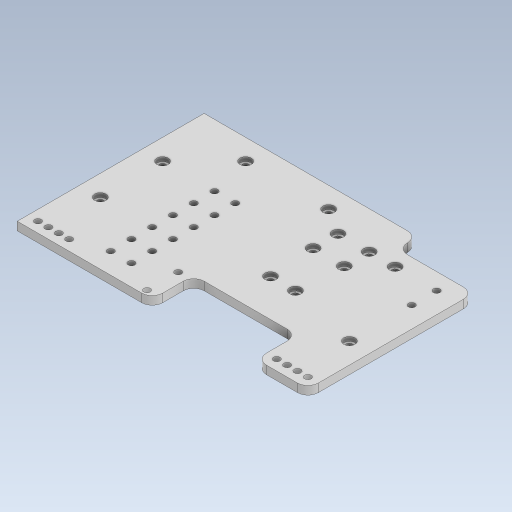
# Autodesk Inventor part: Fix Casis Kiri Belakang
Saved by Autodesk Inventor 2023.5 (Build 275446000, 446)
## iProperties
Created: 2025-10-01
Part Number: Fix Casis Kiri Belakang
Material: Generic
Document SubType Name: Modeling
Designer: Guntur
Density: 1 g/cm^3
Appearance: Default
Author: Guntur
## iProperties of the stored document Fix Casis Kiri Belakang_3DPrint.ipt
Created: 2025-10-18
Part Number: Fix Casis Kiri Belakang_3DPrint
Material: Generic
Document SubType Name: Modeling
Designer: Guntur
Density: 1 g/cm^3
Appearance: Default
Author: Guntur
Autodesk Inventor part; units mm, degrees
ref_plane "YZ Plane" through (0, 0, 0) normal (1, 0, 0) x (0, 1, 0)
ref_plane "XZ Plane" through (0, 0, 0) normal (0, 1, 0) x (-1, 0, 0)
ref_plane "XY Plane" through (0, 0, 0) normal (0, 0, 1) x (1, 0, 0)
sketch "Sketch1" plane through (0, 0, 0) normal (0, 1, 0) x (-1, 0, 0)
  circle A0 centre (-125, -5) radius 1.6
  circle A1 centre (-120, -5) radius 1.6
  line L0 (-115, -20) -> (-115, 0)
  line L1 (-115, 0) -> (-65, 0)
  line L2 (-65, -20) -> (-115, -20)
  line L3 (-65, 0) -> (-65, -20)
  circle A2 centre (-130, -5) radius 1.6
  circle A3 centre (-135, -5) radius 1.6
  circle A4 centre (-82.5, -72) radius 2.75
  line L4 (-140, 0) -> (0, 0)
  line L5 (-140, -90) -> (-140, 0)
  line L6 (0, -90) -> (-140, -90)
  line L7 (0, 0) -> (0, -90)
  circle A5 centre (-10, -30) radius 1.6
  circle A6 centre (-10, -60) radius 1.6
  circle A7 centre (-10, -60) radius 2.75
  circle A8 centre (-10, -30) radius 2.75
  circle A9 centre (-5, -5) radius 1.6
  circle A10 centre (-10, -5) radius 1.6
  circle A11 centre (-15, -5) radius 1.6
  circle A12 centre (-20, -5) radius 1.6
  circle A13 centre (-82.5, -72) radius 1.6
  circle A14 centre (-97.5, -72) radius 1.6
  circle A15 centre (-97.5, -72) radius 2.75
  circle A16 centre (-82.5, -60) radius 1.6
  circle A17 centre (-82.5, -60) radius 2.75
  circle A18 centre (-97.5, -60) radius 1.6
  circle A19 centre (-97.5, -60) radius 2.75
  circle A20 centre (-84, -38) radius 1.6
  circle A21 centre (-84, -38) radius 2.75
  circle A22 centre (-96, -38) radius 1.6
  circle A23 centre (-96, -38) radius 2.75
  circle A24 centre (-130, -30) radius 1.6
  circle A25 centre (-130, -30) radius 2.75
  circle A26 centre (-130, -60) radius 1.6
  circle A27 centre (-130, -60) radius 2.75
  line L8 (-70, -90) -> (-70, 0) construction
  line L9 (0, -45) -> (-140, -45) construction
  circle A28 centre (-125, -85) radius 1.6
  circle A29 centre (-120, -85) radius 1.6
  circle A30 centre (-130, -85) radius 1.6
  circle A31 centre (-135, -85) radius 1.6
  circle A32 centre (-30, -80) radius 1.6
  circle A33 centre (-30, -80) radius 2.75
  circle A34 centre (-70, -80) radius 1.6
  circle A35 centre (-70, -80) radius 2.75
  circle A36 centre (-110, -80) radius 1.6
  circle A37 centre (-110, -80) radius 2.75
  circle A38 centre (-60, -2.5) radius 1.6
  circle A39 centre (-60, -17.5) radius 1.6
  circle A40 centre (-45, -10) radius 1.6
  circle A41 centre (-45, -20) radius 1.6
  circle A42 centre (-35, -20) radius 1.6
  circle A43 centre (-35, -10) radius 1.6
  circle A44 centre (-35, -30) radius 1.6
  circle A45 centre (-35, -40) radius 1.6
  circle A46 centre (-45, -30) radius 1.6
  circle A47 centre (-45, -40) radius 1.6
  circle A48 centre (-35, -50) radius 1.6
  circle A49 centre (-35, -60) radius 1.6
  circle A50 centre (-45, -50) radius 1.6
  circle A51 centre (-45, -60) radius 1.6
  circle A52 centre (-115, -85) radius 1.65
  circle A53 centre (-110, -72) radius 1.6
  circle A54 centre (-110, -72) radius 2.75
  circle A55 centre (-130, -72) radius 1.6
  circle A56 centre (-130, -80) radius 1.6
  line L10 (-140, -90) -> (-103, -90)
  line L11 (-103, -90) -> (-103, -80)
  line L12 (-103, -80) -> (-140, -80)
  line L13 (-140, -80) -> (-140, -90)
  point P0 (-112.75, -80)
  point P1 (-107.25, -80)
  point P2 (-131.6, -80)
  point P3 (-128.4, -80)
  dimension "d29" = 90
  dimension "d30" = 140
  dimension "d31" = 3.2
  dimension "d32" = 30
  dimension "d33" = 10
  dimension "d34" = 5.5
  dimension "d35" = 3.2
  dimension "d36" = 5.5
  dimension "d41" = 10
  dimension "d42" = 10
  dimension "d43" = 10
  dimension "d44" = 10
  dimension "d45" = 10
  dimension "d46" = 3.2
  dimension "d47" = 5
  dimension "d48" = 2.5
  dimension "d49" = 3.2
  dimension "d50" = 15
  dimension "d51" = 3.2
  dimension "d53" = 20
  dimension "d61" = 3.2
  dimension "d62" = 10
  dimension "d63" = 3.2
  dimension "d64" = 10
  dimension "d65" = 3.2
  dimension "d66" = 10
  dimension "d67" = 10
  dimension "d68" = 3.2
  dimension "d69" = 10
  dimension "d70" = 3.2
  dimension "d71" = 10
  dimension "d72" = 3.2
  dimension "d73" = 3.2
  dimension "d74" = 3.2
  dimension "d75" = 10
  dimension "d76" = 3.2
  dimension "d77" = 10
  dimension "d78" = 3.2
  dimension "d79" = 3.2
  dimension "d80" = 3.3
  dimension "d81" = 5
  dimension "d83" = 3.2
  dimension "d84" = 5.5
  dimension "d85" = 3.2
  dimension "d86" = 3.2
  dimension "d87" = 10
  constraints: 57 centre point, 28 end point, 14 coincident, 6 symmetric about line, 3 midpoint, 3 point on line, 2 parallel, 2 perpendicular, 1 horizontal, 6 other
  measures "d29" distance of L6.end L4.start
  measures "d30" distance of L4.start L4.end
  measures "d31" diameter of A32
  measures "d32" distance from line of L7 A32.centre
  measures "d33" distance from line of L6 A32.centre
  measures "d34" diameter of A33
  measures "d35" diameter of A34
  measures "d36" diameter of A35
  measures "d41" distance from line of L6 A34.centre
  measures "d42" distance from line of L7 A7.centre
  measures "d43" distance from line of L7 A5.centre
  measures "d44" distance from line of L5 A27.centre
  measures "d45" distance from line of L5 A25.centre
  measures "d46" diameter of A38
  measures "d47" distance from line of L3 A38.centre
  measures "d48" distance from line of L4 A38.centre
  measures "d49" diameter of A39
  measures "d50" distance of A39.centre A38.centre
  measures "d51" diameter of A40
  measures "d53" distance from line of L3 A40.centre
  measures "d61" diameter of A41
  measures "d62" distance of A41.centre A40.centre
  measures "d63" diameter of A42
  measures "d64" distance of A41.centre A42.centre
  measures "d65" diameter of A43
  measures "d66" distance from line of L4 A40.centre
  measures "d67" distance of A40.centre A43.centre
  measures "d68" diameter of A44
  measures "d69" distance of A44.centre A42.centre
  measures "d70" diameter of A45
  measures "d71" distance of A45.centre A44.centre
  measures "d72" diameter of A46
  measures "d73" diameter of A47
  measures "d74" diameter of A48
  measures "d75" distance of A45.centre A48.centre
  measures "d76" diameter of A49
  measures "d77" distance of A49.centre A48.centre
  measures "d78" diameter of A50
  measures "d79" diameter of A51
  measures "d80" diameter of A52
  measures "d81" distance of A29.centre A52.centre
  measures "d83" diameter of A53
  measures "d84" diameter of A54
  measures "d85" diameter of A55
  measures "d86" diameter of A56
  measures "d87" distance of L10.end L11.end
extrude "Extrusion1" add sketch "Sketch1" along normal blind 4 contours L2 L3 L4 L7 L6 L11 L12 A37 A56 L5 L0 | A56 L12 | A37 L12 A36 | A36 L12 | A27 picked at (-129.8109, -79.5013) picked at (-109.5002, -77.7035) picked at (-109.8109, -79.5013)
extrude "Extrusion2" add sketch "Sketch1" along normal blind 2 contours A4 | A7 | A8 | A15 | A17 | A19 | A21 | A23 | A25 | A27 | A33 | A35 | A54
fillet "Fillet1" radius 5 8 edges at (65, 2, 0) (115, 2, 0) (65, 2, -20) (115, 2, -20) (140, 2, 0) (140, 2, -80) (103, 2, -90) (103, 2, -80)
body "Solid1"
